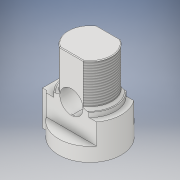
# Autodesk Inventor part: zadnji deo klipa
Saved by Autodesk Inventor 2019 (Build 230136000, 136)
## iProperties
Created: 2018-11-25
Part Number: zadnji deo klipa
Material: ABS Plastic
Document SubType Name: Modeling
Designer: aleks
Density: 1.06 g/cm^3
Appearance: Smooth - White
Author: aleks
Autodesk Inventor part; units mm, degrees
ref_plane "YZ Plane" through (0, 0, 0) normal (1, 0, 0) x (0, 1, 0)
ref_plane "XZ Plane" through (0, 0, 0) normal (0, 1, 0) x (-1, 0, 0)
ref_plane "XY Plane" through (0, 0, 0) normal (0, 0, 1) x (1, 0, 0)
sketch "Sketch1" plane through (0, 0, 0) normal (0, 1, 0) x (-1, 0, 0)
  arc A0 (11.5434, 7) -> (11.5434, -7) centre (0, 0) ccw
  line L0 (13.5, -7) -> (13.5, 7)
  line L1 (13.5, -7) -> (11.5434, -7)
  line L2 (13.5, 7) -> (11.5434, 7)
  dimension "d0" = 27
  dimension "d2" = 14
  constraints: 6 end point, 2 horizontal, 2 point on circle, 1 centre point, 1 coincident
  measures "d0" diameter of A0
  measures "d2" distance of L0.start L0.end
extrude "Extrusion1" add sketch "Sketch1" along normal blind 15
sketch "Sketch2" plane through (0, 15, 0) normal (0, 1, 0) x (1, 0, 0)
  arc A0 (-11.5434, -7) -> (-11.5434, 7) centre (0, 0) ccw projected
  circle A1 centre (0, 0) radius 11
  dimension "d6" = 22
  constraints: 1 centre point, 1 coincident
  measures "d6" diameter of A1
extrude "Extrusion2" add sketch "Sketch2" along normal blind 2
sketch "Sketch3" plane through (0, 17, 0) normal (0, 1, 0) x (1, 0, 0)
  circle A0 centre (0, 0) radius 9.5
  dimension "d9" = 19
  constraints: 1 centre point, 1 coincident
  measures "d9" diameter of A0
extrude "Extrusion3" add sketch "Sketch3" along normal blind 2
fillet "Fillet1" radius 1 1 edges at (-9.5, 17, 0)
sketch "Sketch4" plane through (0, 19, 0) normal (0, 1, 0) x (1, 0, 0)
  circle A0 centre (0, 0) radius 9.5 projected
  circle A1 centre (0, 0) radius 10
  dimension "d13" = 20
  constraints: 1 centre point, 1 coincident
  measures "d13" diameter of A1
extrude "Extrusion4" add sketch "Sketch4" along normal blind 16 contours A0
sketch "Sketch5" plane through (0, 35, 0) normal (0, 1, 0) x (1, 0, 0)
  circle A0 centre (0, 0) radius 9.5 projected
  line L0 (0, 0) -> (8, 0) construction
  line L1 (0, -8) -> (-19.2017, -8)
  line L2 (-19.2017, -8) -> (-19.2017, -21.9067)
  line L3 (-19.2017, -21.9067) -> (19.6427, -21.9067)
  line L4 (19.6427, -21.9067) -> (19.6427, -8)
  line L5 (19.6427, -8) -> (0, -8)
  line L6 (0, 8) -> (-19.2017, 8)
  line L7 (-19.2017, 8) -> (-19.2017, 24.6239)
  line L8 (-19.2017, 24.6239) -> (24.0089, 24.6239)
  line L9 (0, 8) -> (27.6995, 8)
  line L10 (27.6995, 8) -> (27.6995, 24.6239)
  line L11 (27.6995, 24.6239) -> (24.0089, 24.6239)
  constraints: 24 end point, 6 perpendicular, 3 horizontal, 3 point on line, 1 parallel
extrude "Extrusion5" cut sketch "Sketch5" against normal blind 29 contours L9 L6 A0 | A0 L6 L7 L8 L11 L10 L9 | L5 L4 L3 L2 L1 A0 | A0 L1 L5
sketch "Sketch6" plane through (-13.5, 0, -7) normal (-1, 0, 0) x (0, 0, 1)
  circle A0 centre (7, 7.5) radius 4.5
  point P0 (7, 0)
  dimension "d21" = 9
  constraints: 1 centre point
  measures "d21" diameter of A0
extrude "Extrusion6" cut sketch "Sketch6" against normal blind 19
sketch "Sketch7" plane through (0, 0, 0) normal (0, -1, 0) x (1, 0, 0)
  circle A0 centre (0, 0) radius 7.5
  dimension "d26" = 15
  constraints: 1 centre point, 1 coincident
  measures "d26" diameter of A0
extrude "Extrusion7" cut sketch "Sketch7" against normal blind 12
thread "Thread1" size "M10x1" class "6g" standard "ISO Metric profile" full length
thread "Thread2" size "M20x1" class "6g" standard "ISO Metric profile" full length
fillet "Fillet2" radius 0.3 4 edges at (9.5, 35, 0) (-9.5, 35, 0) (0, 35, 8) (0, 35, -8)
thread "Thread3" size "M8x0.8" class "6H" standard "ISO Metric profile" full length
sketch "Sketch8" plane through (-10.8743, 6, 8) normal (0, 0, 1) x (1, 0, 0)
  circle A0 centre (10.8743, 11) radius 5
  point P0 (10.8743, -6)
  dimension "d34" = 10
  constraints: 1 centre point
  measures "d34" diameter of A0
extrude "Extrusion8" cut sketch "Sketch8" against normal blind 20
sketch "Sketch9" plane through (0, 0, 0) normal (0, -1, 0) x (1, 0, 0)
  point P0 (0, 0)
body "Solid1"
